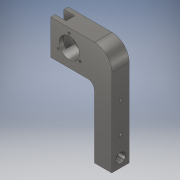
# Autodesk Inventor part: Column
Saved by Autodesk Inventor 2018 (Build 220112000, 112)
## iProperties
Created: 2017-12-19
Part Number: Column
Material: Stainless Steel
Document SubType Name: Modeling
Designer: 232963
Density: 8 g/cm^3
Appearance: Semi-Polished
Author: 232963
Autodesk Inventor part; units mm, degrees
ref_plane "YZ Plane" through (0, 0, 0) normal (1, 0, 0) x (0, 1, 0)
ref_plane "XZ Plane" through (0, 0, 0) normal (0, 1, 0) x (-1, 0, 0)
ref_plane "XY Plane" through (0, 0, 0) normal (0, 0, 1) x (1, 0, 0)
sketch "Sketch1" plane through (0, 0, 0) normal (0, 0, 1) x (1, 0, 0)
  line L0 (63.5, 0) -> (88.9, 0)
  line L1 (88.9, 0) -> (88.9, 127)
  line L2 (63.5, 152.4) -> (0, 152.4)
  line L3 (0, 152.4) -> (0, 101.6)
  line L4 (63.5, 0) -> (63.5, 92.075)
  line L5 (53.975, 101.6) -> (0, 101.6)
  arc A0 (88.9, 127) -> (63.5, 152.4) centre (63.5, 127) ccw
  arc A1 (63.5, 92.075) -> (53.975, 101.6) centre (53.975, 92.075) ccw
  point P0 (0, 0)
  dimension "d2" = 25.4
  dimension "d3" = 50.8
  dimension "d4" = 25.4
  dimension "d5" = 9.525
  constraints: 12 end point, 4 point on circle, 4 tangent, 2 centre point, 2 parallel, 1 horizontal, 1 perpendicular
  measures "d2" distance between parallel lines of L1 L4
  measures "d3" distance between parallel lines of L2 L5
  measures "d4" radius of A0
  measures "d5" radius of A1
extrude "Extrusion1" add sketch "Sketch1" along normal blind 25.4
sketch "Sketch2" plane through (0, 0, 25.4) normal (0, 0, 1) x (1, 0, 0)
  line L0 (63.5, 152.4) -> (0, 152.4) projected
  line L1 (0, 152.4) -> (0, 101.6) projected
  point P0 (0, 0)
  point P1 (26.9748, 127)
  dimension "d8" = 25.4
  dimension "d9" = 26.9748
  measures "d8" distance from line of point (26.975, 127) L0
  measures "d9" distance from line of L1 point (26.975, 127)
hole "Hole1" at (26.9748, 127, 25.4) direction (0, 0, -1) diameter 17.399 end through all counterbore diameter 29.718 counterbore depth 19.7104
sketch "Sketch3" plane through (0, 0, 25.4) normal (0, 0, 1) x (1, 0, 0)
  line L0 (0, 152.4) -> (0, 101.6) projected
  circle A0 centre (26.9748, 127) radius 14.859 projected
  point P0 (0, 0)
  point P1 (26.9748, 145.415)
  dimension "d17" = 26.9748
  dimension "d18" = 18.415
  measures "d17" distance from line of L0 point (26.975, 145.415)
  measures "d18" distance of A0.centre point (26.975, 145.415)
hole "Hole2" at (26.9748, 145.415, 25.4) direction (0, 0, -1) diameter 3.302 depth 9.525 tip angle 118 thread size "8-32 UNC" class "2B" standard "ANSI Unified Screw Threads"
pattern_circular "Circular Pattern1" count 3 over 360 about axis through (26.9748, 127, 15.5448) along (0, 0, 1) of "Hole2"
sketch "Sketch4" plane through (0, 101.6, 0) normal (-1, 0, 0) x (0, 0, 1)
  line L0 (0, 50.8) -> (25.4, 50.8) projected
  line L1 (0, 0) -> (25.4, 0) projected
  line L2 (25.4, 50.8) -> (25.4, 0) projected
  line L3 (0, 0) -> (0, 50.8) projected
  line L4 (6.35, 0) -> (19.05, 0)
  line L5 (19.05, 0) -> (19.05, 50.8)
  line L6 (19.05, 50.8) -> (6.35, 50.8)
  line L7 (6.35, 50.8) -> (6.35, 0)
  point P0 (0, -101.6)
  dimension "d31" = 6.35
  dimension "d32" = 6.35
  constraints: 8 end point, 2 parallel, 2 point on line, 1 horizontal, 1 perpendicular
  measures "d31" distance between parallel lines of L3 L7
  measures "d32" distance between parallel lines of L2 L5
extrude "Extrusion2" cut sketch "Sketch4" against normal blind 15.875 contours L0 L5 L1 L7
sketch "Sketch5" plane through (0, 101.6, 0) normal (-1, 0, 0) x (0, 0, 1)
  line L0 (0, 50.8) -> (6.35, 50.8) projected
  line L1 (0, 0) -> (0, 50.8) projected
  point P0 (0, -101.6)
  point P1 (3.175, 47.625)
  dimension "d35" = 3.175
  dimension "d36" = 3.175
  measures "d35" distance from line of L0 point (3.175, 47.625)
  measures "d36" distance from line of L1 point (3.175, 47.625)
hole "Hole3" at (0, 149.225, 3.175) direction (1, 0, 0) diameter 3.302 depth 11.1252 tip angle 118 thread size "8-32 UNC" class "2B" standard "ANSI Unified Screw Threads"
pattern_linear "Rectangular Pattern1" count 2 spacing 19.05 along (0, 0, 1) count 2 spacing 44.45 along (0, -1, 0) of "Hole3"
sketch "Sketch6" plane through (63.5, 0, 0) normal (-1, 0, 0) x (0, 0, 1)
  line L0 (0, 0) -> (0, 92.075) projected
  line L1 (0, 0) -> (25.4, 0) projected
  point P0 (12.7, 85.09)
  point P1 (12.7, 41.91)
  dimension "d50" = 43.18
  dimension "d51" = 12.7
  dimension "d52" = 12.7
  dimension "d53" = 41.91
  measures "d50" distance of point (12.7, 85.09) point (12.7, 41.91)
  measures "d51" distance from line of L0 point (12.7, 85.09)
  measures "d52" distance from line of L0 point (12.7, 41.91)
  measures "d53" distance from line of L1 point (12.7, 41.91)
hole "Hole4" at (63.5, 85.09, 12.7) at (63.5, 41.91, 12.7) direction (1, 0, 0) diameter 4.3688 end through all countersink diameter 9.525 countersink angle 82
sketch "Sketch7" plane through (88.9, 0, 0) normal (1, 0, 0) x (0, 0, -1)
  line L0 (0, 0) -> (-25.4, 0) projected
  line L1 (0, 127) -> (0, 0) projected
  point P0 (-12.7, 12.7)
  dimension "d61" = 12.7
  dimension "d62" = 12.7
  measures "d61" distance from line of L0 point (-12.7, 12.7)
  measures "d62" distance from line of L1 point (-12.7, 12.7)
hole "Hole5" at (88.9, 12.7, 12.7) direction (-1, 0, 0) diameter 9.906 end through all counterbore diameter 14.2748 counterbore depth 9.525
sketch "Sketch8" plane through (0, 0, 0) normal (0, 0, -1) x (-1, 0, 0)
  line L0 (0, 152.4) -> (-63.5, 152.4) projected
  line L1 (0, 101.6) -> (0, 152.4) projected
  point P0 (0, 0)
  point P1 (-39.6748, 127)
  point P2 (-14.2748, 127)
  dimension "d70" = 25.4
  dimension "d71" = 25.4
  dimension "d72" = 14.2748
  dimension "d73" = 39.6748
  measures "d70" distance from line of L0 point (-39.675, 127)
  measures "d71" distance from line of L0 point (-14.275, 127)
  measures "d72" distance from line of L1 point (-14.275, 127)
  measures "d73" distance from line of L1 point (-39.675, 127)
hole "Hole6" at (39.6748, 127, 0) at (14.2748, 127, 0) direction (0, 0, 1) diameter 3.302 depth 6.35 tip angle 118 thread size "8-32 UNC" class "2B" standard "ANSI Unified Screw Threads"
body "Solid1"
